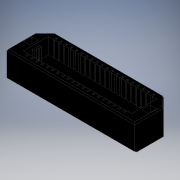
# Autodesk Inventor part: QTE-020-01-Dt
Saved by Autodesk Inventor 2019 (Build 230136000, 136)
## iProperties
Created: 2024-08-20
Part Number: QTE-020-01-Dt
Material: Generic
Catalog Web Link: www.cadenas.de
Description: QTE Series Terminal-QTE Series - (0,80 mm) .0315" Q Strip® High Speed Ground Plane Header
Vendor: SAMTEC
Document SubType Name: Modeling
Designer: psAdmin
Manufacturer: SAMTEC
Mass: 0.287371 g
Surface Area: 6.67562 cm^2
Volume: 0.287371 cm^3
Density: 1 g/cm^3
Appearance: PSOLRGB-14-14-14
Category: PARTsolutions
Company: SAMTEC
Title: QTE-020-01-Dt
Author: Cadenas PARTsolutions
Comments: QTE Series - (0,80 mm) .0315" Q Strip® High Speed Ground Plane Header
PSOL_IDENT_0: {$CADENAS_DATA/23d-libs/samtec/modelling/qte/parts/qte_terminal.prj},235 {VTYP=3D},{NB=QTE-020-01-Dt
PSOL_IDENT_1: },{LINA=QTE-020-01-Dt},{NN=QTE Series Terminal},{DATE=15.07.2024 08:39:37},{GEOMDATE=05.07.2024 10:0
PSOL_IDENT_2: 5:00},{VERSION=},{LINEID=20},{WBVAR=POS,LS,ROW,AOPT,LCOPT,GPOPT,SDOPT,FLOPT,RT1OPT,LOPT,KOPT},{WBNUM
PSOL_IDENT_3: ERIC=}  {NB=QTE-020-01-Dt},{LINA=QTE-020-01-Dt},{KT=DUMMY},{PN=QTE-020-01-D},{SERIES=QTE},{MP=0},{PO
PSOL_IDENT_4: S=020},{LS=01},{SL=0.66850},{ROW=D},{AOPT=},{LCOPT=},{GPOPT=},{SDOPT=},{FLOPT=},{RT1OPT=},{LOPT=},{K
PSOL_IDENT_5: OPT=},{AW=0.78800},{FGP=1.01300},{A=0.16800},{D=0.72800},{X=0.0930},{Z=0.59850},{DX=0.00000},{CH=0.1
PSOL_IDENT_6: 6000},{N=0.85400},{K=0.91500},{SP=0.76450},{BBH=0.00000},{EGP=1.30500},{HGP=0.36300},{GRT1=1.43800},
PSOL_IDENT_7: {HRT1=1.12900},{TKOPT=0.17300},{X1DP=0.00000},{AOPTPN=},{ROWALG= 'D','-D - Double' },{LCOPTALG= '','
PSOL_IDENT_8: Not Selected','LC','-LC - Locking Clips' },{LCOPTPN=},{GPOPTALG= '','Not Selected','GP','-GP - Guide
PSOL_IDENT_9: Posts' },{GPOPTPN=},{SDOPTALG= '','Not Selected','SD','-SD - Screw Down' },{SDOPTPN=},{FLOPTALG= ''
PSOL_IDENT_10: ,'Not Selected','FL','-FL - Friction Locks' },{FLOPTPN=},{RT1OPTALG= '','Not Available' },{RT1OPTPN=
PSOL_IDENT_11: },{LOPTALG= '','Not Available' },{LOPTPN=},{KOPTALG= '','Not Selected','K','-K - Polyimide Film' },{
PSOL_IDENT_12: KOPTPN=},{TROPTALG= '','Not Selected','TR','-TR - Tape & Reel' }
NB: QTE-020-01-Dt
NN: QTE Series Terminal
NT: QTE Series - (0,80 mm) .0315" Q Strip® High Speed Ground Plane Header
NBSYN: $PN.t
LINA: QTE-020-01-Dt
CATALOG: Samtec
PN: QTE-020-01-D
SERIES: QTE
MP: 0
POS: 020
LS: -01
SL: 0.6685
ROW: -D - Double
AOPT: Not Selected
LCOPT: Not Selected
GPOPT: Not Selected
SDOPT: Not Selected
FLOPT: Not Selected
RT1OPT: Not Available
LOPT: Not Available
KOPT: Not Selected
AW: 0.788
FGP: 1.013
A: 0.168
D: 0.728
X: 0.093
Z: 0.5985
DX: 0
CH: 0.16
N: 0.854
K: 0.915
SP: 0.7645
BBH: 0
EGP: 1.305
HGP: 0.363
GRT1: 1.438
HRT1: 1.129
TKOPT: 0.173
X1DP: 0
SUPPLIER: SAMTEC
ARTICLENO: QTE-020-01-Dt
BOMINFO: QTE-020-01-Dt
CREATOR: CADENAS GmbH
Autodesk Inventor part; units mm, degrees
sketch "Sketch_1" plane through (0, 0, 0) normal (0, 1, 0) x (-1, 0, 0)
  line L0 (10.0076, 2.9845) -> (-10.0076, 2.9845)
  line L1 (-10.0076, 2.9845) -> (-10.0076, -1.4605)
  line L2 (-10.0076, -1.4605) -> (-8.4836, -2.9845)
  line L3 (-8.4836, -2.9845) -> (8.4836, -2.9845)
  line L4 (8.4836, -2.9845) -> (10.0076, -1.4605)
  line L5 (10.0076, -1.4605) -> (10.0076, 2.9845)
  constraints: 12 end point
extrude "Extrusion1" add sketch "Sketch_1" along normal blind 3.81
sketch "Sketch_7" plane through (0, 3.81, 0) normal (0, 1, 0) x (1, 0, 0)
  line L0 (-10.0076, -2.9845) -> (10.0076, -2.9845)
  line L1 (10.0076, -2.9845) -> (10.0076, 1.4605)
  line L2 (10.0076, 1.4605) -> (8.4836, 2.9845)
  line L3 (8.4836, 2.9845) -> (-8.4836, 2.9845)
  line L4 (-8.4836, 2.9845) -> (-10.0076, 1.4605)
  line L5 (-10.0076, 1.4605) -> (-10.0076, -2.9845)
  constraints: 12 end point
extrude "Extrusion2" add sketch "Sketch_7" along normal blind 0.254 draft -30.964
sketch "Sketch_16" plane through (0, 4.064, 0) normal (0, 1, 0) x (1, 0, 0)
  line L0 (-8.4582, 1.9685) -> (-8.4582, -1.9685)
  line L1 (-8.4582, -1.9685) -> (-7.6898, -1.9685)
  line L2 (-7.6898, -1.9685) -> (-7.6898, -2.4003)
  line L3 (-7.6898, -2.4003) -> (-7.474, -2.4003)
  line L4 (-7.474, -2.4003) -> (-7.474, -1.9685)
  line L5 (-7.474, -1.9685) -> (-6.8898, -1.9685)
  line L6 (-6.8898, -1.9685) -> (-6.8898, -2.4003)
  line L7 (-6.8898, -2.4003) -> (-6.6738, -2.4003)
  line L8 (-6.6738, -2.4003) -> (-6.6738, -1.9685)
  line L9 (-6.6738, -1.9685) -> (-6.0896, -1.9685)
  line L10 (-6.0896, -1.9685) -> (-6.0896, -2.4003)
  line L11 (-6.0896, -2.4003) -> (-5.8738, -2.4003)
  line L12 (-5.8738, -2.4003) -> (-5.8738, -1.9685)
  line L13 (-5.8738, -1.9685) -> (-5.2895, -1.9685)
  line L14 (-5.2895, -1.9685) -> (-5.2895, -2.4003)
  line L15 (-5.2895, -2.4003) -> (-5.0737, -2.4003)
  line L16 (-5.0737, -2.4003) -> (-5.0737, -1.9685)
  line L17 (-5.0737, -1.9685) -> (-4.4894, -1.9685)
  line L18 (-4.4894, -1.9685) -> (-4.4894, -2.4003)
  line L19 (-4.4894, -2.4003) -> (-4.2736, -2.4003)
  line L20 (-4.2736, -2.4003) -> (-4.2736, -1.9685)
  line L21 (-4.2736, -1.9685) -> (-3.6893, -1.9685)
  line L22 (-3.6893, -1.9685) -> (-3.6893, -2.4003)
  line L23 (-3.6893, -2.4003) -> (-3.4735, -2.4003)
  line L24 (-3.4735, -2.4003) -> (-3.4735, -1.9685)
  line L25 (-3.4735, -1.9685) -> (-2.8892, -1.9685)
  line L26 (-2.8892, -1.9685) -> (-2.8892, -2.4003)
  line L27 (-2.8892, -2.4003) -> (-2.6734, -2.4003)
  line L28 (-2.6734, -2.4003) -> (-2.6734, -1.9685)
  line L29 (-2.6734, -1.9685) -> (-2.0892, -1.9685)
  line L30 (-2.0892, -1.9685) -> (-2.0892, -2.4003)
  line L31 (-2.0892, -2.4003) -> (-1.8732, -2.4003)
  line L32 (-1.8732, -2.4003) -> (-1.8732, -1.9685)
  line L33 (-1.8732, -1.9685) -> (-1.2891, -1.9685)
  line L34 (-1.2891, -1.9685) -> (-1.2891, -2.4003)
  line L35 (-1.2891, -2.4003) -> (-1.0732, -2.4003)
  line L36 (-1.0732, -2.4003) -> (-1.0732, -1.9685)
  line L37 (-1.0732, -1.9685) -> (-0.489, -1.9685)
  line L38 (-0.489, -1.9685) -> (-0.489, -2.4003)
  line L39 (-0.489, -2.4003) -> (-0.2731, -2.4003)
  line L40 (-0.2731, -2.4003) -> (-0.2731, -1.9685)
  line L41 (-0.2731, -1.9685) -> (0.3111, -1.9685)
  line L42 (0.3111, -1.9685) -> (0.3111, -2.4003)
  line L43 (0.3111, -2.4003) -> (0.5271, -2.4003)
  line L44 (0.5271, -2.4003) -> (0.5271, -1.9685)
  line L45 (0.5271, -1.9685) -> (1.1112, -1.9685)
  line L46 (1.1112, -1.9685) -> (1.1112, -2.4003)
  line L47 (1.1112, -2.4003) -> (1.3272, -2.4003)
  line L48 (1.3272, -2.4003) -> (1.3272, -1.9685)
  line L49 (1.3272, -1.9685) -> (1.9114, -1.9685)
  line L50 (1.9114, -1.9685) -> (1.9114, -2.4003)
  line L51 (1.9114, -2.4003) -> (2.1273, -2.4003)
  line L52 (2.1273, -2.4003) -> (2.1273, -1.9685)
  line L53 (2.1273, -1.9685) -> (2.7115, -1.9685)
  line L54 (2.7115, -1.9685) -> (2.7115, -2.4003)
  line L55 (2.7115, -2.4003) -> (2.9274, -2.4003)
  line L56 (2.9274, -2.4003) -> (2.9274, -1.9685)
  line L57 (2.9274, -1.9685) -> (3.5116, -1.9685)
  line L58 (3.5116, -1.9685) -> (3.5116, -2.4003)
  line L59 (3.5116, -2.4003) -> (3.7275, -2.4003)
  line L60 (3.7275, -2.4003) -> (3.7275, -1.9685)
  line L61 (3.7275, -1.9685) -> (4.3117, -1.9685)
  line L62 (4.3117, -1.9685) -> (4.3117, -2.4003)
  line L63 (4.3117, -2.4003) -> (4.5275, -2.4003)
  line L64 (4.5275, -2.4003) -> (4.5275, -1.9685)
  line L65 (4.5275, -1.9685) -> (5.1118, -1.9685)
  line L66 (5.1118, -1.9685) -> (5.1118, -2.4003)
  line L67 (5.1118, -2.4003) -> (5.3276, -2.4003)
  line L68 (5.3276, -2.4003) -> (5.3276, -1.9685)
  line L69 (5.3276, -1.9685) -> (5.9119, -1.9685)
  line L70 (5.9119, -1.9685) -> (5.9119, -2.4003)
  line L71 (5.9119, -2.4003) -> (6.1277, -2.4003)
  line L72 (6.1277, -2.4003) -> (6.1277, -1.9685)
  line L73 (6.1277, -1.9685) -> (6.7119, -1.9685)
  line L74 (6.7119, -1.9685) -> (6.7119, -2.4003)
  line L75 (6.7119, -2.4003) -> (6.9278, -2.4003)
  line L76 (6.9278, -2.4003) -> (6.9278, -1.9685)
  line L77 (6.9278, -1.9685) -> (7.5121, -1.9685)
  line L78 (7.5121, -1.9685) -> (7.5121, -2.4003)
  line L79 (7.5121, -2.4003) -> (7.7279, -2.4003)
  line L80 (7.7279, -2.4003) -> (7.7279, -1.9685)
  line L81 (7.7279, -1.9685) -> (8.4582, -1.9685)
  line L82 (8.4582, -1.9685) -> (8.4582, 1.9685)
  line L83 (8.4582, 1.9685) -> (7.7279, 1.9685)
  line L84 (7.7279, 1.9685) -> (7.7279, 2.4003)
  line L85 (7.7279, 2.4003) -> (7.5121, 2.4003)
  line L86 (7.5121, 2.4003) -> (7.5121, 1.9685)
  line L87 (7.5121, 1.9685) -> (6.9278, 1.9685)
  line L88 (6.9278, 1.9685) -> (6.9278, 2.4003)
  line L89 (6.9278, 2.4003) -> (6.7119, 2.4003)
  line L90 (6.7119, 2.4003) -> (6.7119, 1.9685)
  line L91 (6.7119, 1.9685) -> (6.1277, 1.9685)
  line L92 (6.1277, 1.9685) -> (6.1277, 2.4003)
  line L93 (6.1277, 2.4003) -> (5.9119, 2.4003)
  line L94 (5.9119, 2.4003) -> (5.9119, 1.9685)
  line L95 (5.9119, 1.9685) -> (5.3276, 1.9685)
  line L96 (5.3276, 1.9685) -> (5.3276, 2.4003)
  line L97 (5.3276, 2.4003) -> (5.1118, 2.4003)
  line L98 (5.1118, 2.4003) -> (5.1118, 1.9685)
  line L99 (5.1118, 1.9685) -> (4.5275, 1.9685)
  line L100 (4.5275, 1.9685) -> (4.5275, 2.4003)
  line L101 (4.5275, 2.4003) -> (4.3117, 2.4003)
  line L102 (4.3117, 2.4003) -> (4.3117, 1.9685)
  line L103 (4.3117, 1.9685) -> (3.7275, 1.9685)
  line L104 (3.7275, 1.9685) -> (3.7275, 2.4003)
  line L105 (3.7275, 2.4003) -> (3.5116, 2.4003)
  line L106 (3.5116, 2.4003) -> (3.5116, 1.9685)
  line L107 (3.5116, 1.9685) -> (2.9274, 1.9685)
  line L108 (2.9274, 1.9685) -> (2.9274, 2.4003)
  line L109 (2.9274, 2.4003) -> (2.7115, 2.4003)
  line L110 (2.7115, 2.4003) -> (2.7115, 1.9685)
  line L111 (2.7115, 1.9685) -> (2.1273, 1.9685)
  line L112 (2.1273, 1.9685) -> (2.1273, 2.4003)
  line L113 (2.1273, 2.4003) -> (1.9114, 2.4003)
  line L114 (1.9114, 2.4003) -> (1.9114, 1.9685)
  line L115 (1.9114, 1.9685) -> (1.3272, 1.9685)
  line L116 (1.3272, 1.9685) -> (1.3272, 2.4003)
  line L117 (1.3272, 2.4003) -> (1.1112, 2.4003)
  line L118 (1.1112, 2.4003) -> (1.1112, 1.9685)
  line L119 (1.1112, 1.9685) -> (0.5271, 1.9685)
  line L120 (0.5271, 1.9685) -> (0.5271, 2.4003)
  line L121 (0.5271, 2.4003) -> (0.3111, 2.4003)
  line L122 (0.3111, 2.4003) -> (0.3111, 1.9685)
  line L123 (0.3111, 1.9685) -> (-0.2731, 1.9685)
  line L124 (-0.2731, 1.9685) -> (-0.2731, 2.4003)
  line L125 (-0.2731, 2.4003) -> (-0.489, 2.4003)
  line L126 (-0.489, 2.4003) -> (-0.489, 1.9685)
  line L127 (-0.489, 1.9685) -> (-1.0732, 1.9685)
  line L128 (-1.0732, 1.9685) -> (-1.0732, 2.4003)
  line L129 (-1.0732, 2.4003) -> (-1.2891, 2.4003)
  line L130 (-1.2891, 2.4003) -> (-1.2891, 1.9685)
  line L131 (-1.2891, 1.9685) -> (-1.8732, 1.9685)
  line L132 (-1.8732, 1.9685) -> (-1.8732, 2.4003)
  line L133 (-1.8732, 2.4003) -> (-2.0892, 2.4003)
  line L134 (-2.0892, 2.4003) -> (-2.0892, 1.9685)
  line L135 (-2.0892, 1.9685) -> (-2.6734, 1.9685)
  line L136 (-2.6734, 1.9685) -> (-2.6734, 2.4003)
  line L137 (-2.6734, 2.4003) -> (-2.8892, 2.4003)
  line L138 (-2.8892, 2.4003) -> (-2.8892, 1.9685)
  line L139 (-2.8892, 1.9685) -> (-3.4735, 1.9685)
  line L140 (-3.4735, 1.9685) -> (-3.4735, 2.4003)
  line L141 (-3.4735, 2.4003) -> (-3.6893, 2.4003)
  line L142 (-3.6893, 2.4003) -> (-3.6893, 1.9685)
  line L143 (-3.6893, 1.9685) -> (-4.2736, 1.9685)
  line L144 (-4.2736, 1.9685) -> (-4.2736, 2.4003)
  line L145 (-4.2736, 2.4003) -> (-4.4894, 2.4003)
  line L146 (-4.4894, 2.4003) -> (-4.4894, 1.9685)
  line L147 (-4.4894, 1.9685) -> (-5.0737, 1.9685)
  line L148 (-5.0737, 1.9685) -> (-5.0737, 2.4003)
  line L149 (-5.0737, 2.4003) -> (-5.2895, 2.4003)
  line L150 (-5.2895, 2.4003) -> (-5.2895, 1.9685)
  line L151 (-5.2895, 1.9685) -> (-5.8738, 1.9685)
  line L152 (-5.8738, 1.9685) -> (-5.8738, 2.4003)
  line L153 (-5.8738, 2.4003) -> (-6.0896, 2.4003)
  line L154 (-6.0896, 2.4003) -> (-6.0896, 1.9685)
  line L155 (-6.0896, 1.9685) -> (-6.6738, 1.9685)
  line L156 (-6.6738, 1.9685) -> (-6.6738, 2.4003)
  line L157 (-6.6738, 2.4003) -> (-6.8898, 2.4003)
  line L158 (-6.8898, 2.4003) -> (-6.8898, 1.9685)
  line L159 (-6.8898, 1.9685) -> (-7.474, 1.9685)
  line L160 (-7.474, 1.9685) -> (-7.474, 2.4003)
  line L161 (-7.474, 2.4003) -> (-7.6898, 2.4003)
  line L162 (-7.6898, 2.4003) -> (-7.6898, 1.9685)
  line L163 (-7.6898, 1.9685) -> (-8.4582, 1.9685)
  constraints: 328 end point
extrude "Extrusion3" cut sketch "Sketch_16" along normal mid plane 4.9784
sketch "Sketch_32" plane through (0, 0, 0) normal (0, 1, 0) x (-1, 0, 0)
  line L0 (9.7536, -0.635) -> (9.7536, 0.635)
  line L1 (9.7536, 0.635) -> (8.7376, 0.635)
  line L2 (8.7376, 0.635) -> (8.7376, -0.635)
  line L3 (8.7376, -0.635) -> (9.7536, -0.635)
  constraints: 8 end point
extrude "Extrusion4" cut sketch "Sketch_32" along normal mid plane 8.128
sketch "Sketch_33" plane through (0, 0, 0) normal (0, 1, 0) x (-1, 0, 0)
  line L0 (-8.7376, -0.635) -> (-8.7376, 0.635)
  line L1 (-8.7376, 0.635) -> (-9.7536, 0.635)
  line L2 (-9.7536, 0.635) -> (-9.7536, -0.635)
  line L3 (-9.7536, -0.635) -> (-8.7376, -0.635)
  constraints: 8 end point
extrude "Extrusion5" cut sketch "Sketch_33" along normal mid plane 8.128
sketch "Sketch_34" plane through (0, 1.5748, 0) normal (0, 1, 0) x (1, 0, 0)
  line L0 (-8.4963, 0.5715) -> (-8.4963, -0.5715)
  line L1 (-8.4963, -0.5715) -> (-8.0797, -0.5715)
  line L2 (-8.0797, -0.5715) -> (-8.0797, -0.2032)
  line L3 (-8.0797, -0.2032) -> (-8.2067, -0.2032)
  line L4 (-8.2067, -0.2032) -> (-8.2067, 0.2032)
  line L5 (-8.2067, 0.2032) -> (-8.0797, 0.2032)
  line L6 (-8.0797, 0.2032) -> (-8.0797, 0.5715)
  line L7 (-8.0797, 0.5715) -> (-8.4963, 0.5715)
  constraints: 16 end point
extrude "Extrusion6" add sketch "Sketch_34" along normal blind 1.9812
sketch "Sketch_35" plane through (0, 1.5748, 0) normal (0, 1, 0) x (1, 0, 0)
  line L0 (8.1559, 0.2032) -> (8.2829, 0.2032)
  line L1 (8.2829, 0.2032) -> (8.2829, -0.2032)
  line L2 (8.2829, -0.2032) -> (8.1559, -0.2032)
  line L3 (8.1559, -0.2032) -> (8.1559, -0.5715)
  line L4 (8.1559, -0.5715) -> (8.5725, -0.5715)
  line L5 (8.5725, -0.5715) -> (8.5725, 0.5715)
  line L6 (8.5725, 0.5715) -> (8.1559, 0.5715)
  line L7 (8.1559, 0.5715) -> (8.1559, 0.2032)
  constraints: 16 end point
extrude "Extrusion7" add sketch "Sketch_35" along normal blind 1.9812
sketch "Sketch_44" plane through (0, 0, 0) normal (0, 1, 0) x (-1, 0, 0)
  line L0 (9.3726, -0.1905) -> (9.3726, 0.1905)
  line L1 (9.3726, 0.1905) -> (-9.3726, 0.1905)
  line L2 (-9.3726, 0.1905) -> (-9.3726, -0.1905)
  line L3 (-9.3726, -0.1905) -> (9.3726, -0.1905)
  constraints: 8 end point
extrude "Extrusion8" cut sketch "Sketch_44" along normal blind 0.2794
sketch "Sketch_54" plane through (0, 0, 0) normal (1, 0, 0) x (0, 1, 0)
  line L0 (-4.8222, 10) -> (-4.8222, -10)
  line L1 (-4.8222, -10) -> (0.1778, -10)
  line L2 (0.1778, -10) -> (0.1778, -2.7305)
  line L3 (0.1778, -2.7305) -> (0, -2.7305)
  line L4 (0, -2.7305) -> (0, -8.73)
  line L5 (0, -8.73) -> (-3.5522, -8.73)
  line L6 (-3.5522, -8.73) -> (-3.5522, 8.73)
  line L7 (-3.5522, 8.73) -> (0, 8.73)
  line L8 (0, 8.73) -> (0, 2.7305)
  line L9 (0, 2.7305) -> (0.1778, 2.7305)
  line L10 (0.1778, 2.7305) -> (0.1778, 10)
  line L11 (0.1778, 10) -> (-4.8222, 10)
  constraints: 24 end point
extrude "Extrusion9" cut sketch "Sketch_54" along normal mid plane 45.1104
ref_plane "metal_plane_1_XY" through (0, -0.2032, 0) normal (0, 1, 0) x (1, 0, 0)
ref_plane "metal_plane_1_YZ" through (0, -0.2032, 0) normal (1, 0, 0) x (0, 0, -1)
ref_plane "metal_plane_1_ZX" through (0, -0.2032, 0) normal (0, 0, -1) x (0, 1, 0)
ref_plane "pad_1_XY" through (0, 4.064, 0) normal (0, 1, 0) x (1, 0, 0)
ref_plane "pad_1_YZ" through (0, 4.064, 0) normal (1, 0, 0) x (0, 0, -1)
ref_plane "pad_1_ZX" through (0, 4.064, 0) normal (0, 0, -1) x (0, 1, 0)
ref_plane "pin_left_1_XY" through (-7.7407, 0.1778, 3.556) normal (0, 1, 0) x (1, 0, 0)
ref_plane "pin_left_1_YZ" through (-7.7407, 0.1778, 3.556) normal (1, 0, 0) x (0, 0, -1)
ref_plane "pin_left_1_ZX" through (-7.7407, 0.1778, 3.556) normal (0, 0, -1) x (0, 1, 0)
ref_plane "terminal_XY" through (0, 0, 0) normal (0, 1, 0) x (1, 0, 0)
ref_plane "terminal_YZ" through (0, 0, 0) normal (1, 0, 0) x (0, 0, -1)
ref_plane "terminal_ZX" through (0, 0, 0) normal (0, 0, -1) x (0, 1, 0)
body "Solid1"
